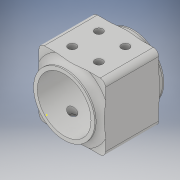
# Autodesk Inventor part: Крепление манипулятора
Saved by Autodesk Inventor 2019.1 (Build 231200000, 200)
## iProperties
Created: 2018-08-01
Part Number: Крепление манипулятора
Material: Типовые
Document SubType Name: Modeling
Designer: olege
Density: 1 g/cm^3
Appearance: По умолчанию
Author: olege
Autodesk Inventor part; units mm, degrees
ref_plane "YZ Plane" through (0, 0, 0) normal (1, 0, 0) x (0, 1, 0)
ref_plane "XZ Plane" through (0, 0, 0) normal (0, 1, 0) x (-1, 0, 0)
sketch "Эскиз1" plane through (0, 0, 0) normal (0, 0, 1) x (1, 0, 0)
  circle A0 centre (0, 0) radius 9.975
  dimension "d0" = 19.95
  constraints: 1 centre point, 1 coincident
  measures "d0" diameter of A0
extrude "Выдавливание1" add sketch "Эскиз1" along normal blind 7.1
sketch "Эскиз2" plane through (0, 0, 7.1) normal (0, 0, 1) x (1, 0, 0)
  circle A0 centre (0, 0) radius 9.975 projected
  circle A1 centre (0, 0) radius 11.5
  dimension "d3" = 23
  constraints: 1 centre point, 1 coincident
  measures "d3" diameter of A1
extrude "Выдавливание2" add sketch "Эскиз2" along normal blind 2.45 contours A0 | A1
sketch "Эскиз3" plane through (0, 0, 9.55) normal (0, 0, 1) x (1, 0, 0)
  line L0 (12.5, 12.5) -> (-12.5, 12.5)
  line L1 (-12.5, 12.5) -> (-12.5, -12.5)
  line L2 (-12.5, -12.5) -> (12.5, -12.5)
  line L3 (12.5, -12.5) -> (12.5, 12.5)
  line L4 (12.5, 12.5) -> (-12.5, -12.5) construction
  line L5 (-12.5, 12.5) -> (12.5, -12.5) construction
  point P0 (0, 0)
  dimension "d6" = 25
  dimension "d7" = 25
  constraints: 12 end point, 2 midpoint, 2 parallel, 1 horizontal, 1 perpendicular
  measures "d6" distance of L2.end L1.end
  measures "d7" distance of L1.end L0.end
extrude "Выдавливание3" add sketch "Эскиз3" along normal blind 20
fillet "Сопряжение1" radius 2.5 1 edges at (-11.5, 0, 9.55)
sketch "Эскиз4" plane through (0, 0, 29.55) normal (0, 0, 1) x (1, 0, 0)
  circle A0 centre (0, 0) radius 11.5
  dimension "d12" = 23
  constraints: 1 centre point, 1 coincident
  measures "d12" diameter of A0
extrude "Выдавливание4" add sketch "Эскиз4" along normal blind 2.5
sketch "Эскиз5" plane through (0, 0, 32.05) normal (0, 0, 1) x (1, 0, 0)
  circle A0 centre (0, 0) radius 9.975
  dimension "d15" = 19.95
  constraints: 1 centre point, 1 coincident
  measures "d15" diameter of A0
extrude "Выдавливание5" add sketch "Эскиз5" along normal blind 7.1
fillet "Сопряжение3" radius 2.5 1 edges at (-11.5, 0, 29.55)
fillet "Сопряжение4" radius 2 4 edges at (-12.5, -12.5, 19.55) (-12.5, 12.5, 19.55) (12.5, 12.5, 19.55) (12.5, -12.5, 19.55)
sketch "Эскиз6" plane through (0, 0, 39.15) normal (0, 0, 1) x (1, 0, 0)
  line L0 (-4, -4) -> (4, -4)
  line L1 (4, -4) -> (4, 4)
  line L2 (4, 4) -> (-4, 4)
  line L3 (-4, 4) -> (-4, -4)
  line L4 (-4, -4) -> (4, 4) construction
  line L5 (4, -4) -> (-4, 4) construction
  point P0 (0, 0)
  dimension "d20" = 8
  dimension "d21" = 8
  constraints: 12 end point, 2 midpoint, 2 parallel, 1 horizontal, 1 perpendicular
  measures "d20" distance of L2.end L1.end
  measures "d21" distance of L1.end L0.end
extrude "Выдавливание6" cut sketch "Эскиз6" against normal blind 8
sketch "Эскиз7" plane through (0, 0, 31.15) normal (0, 0, 1) x (1, 0, 0)
  circle A0 centre (0, 0) radius 1.25
  dimension "d24" = 2.5
  constraints: 1 centre point, 1 coincident
  measures "d24" diameter of A0
extrude "Выдавливание7" cut sketch "Эскиз7" against normal blind 6
sketch "Эскиз8" plane through (0, 0, 0) normal (0, 0, -1) x (-1, 0, 0)
  circle A0 centre (0, 7.5) radius 1.25
  circle A1 centre (0, -7.5) radius 1.25
  point P0 (0, 0)
  dimension "d27" = 2.5
  dimension "d28" = 2.5
  dimension "d29" = 7.5
  dimension "d30" = 7.5
  constraints: 2 centre point, 2 vertical alignment
  measures "d27" diameter of A0
  measures "d28" diameter of A1
  measures "d29" distance of point (0, 0) A1.centre
  measures "d30" distance of point (0, 0) A0.centre
extrude "Выдавливание8" cut sketch "Эскиз8" against normal blind 12
ref_plane "РабПлоскость1" through (-5.6789, -12.5, 7.55) normal (0, -1, 0) x (1, 0, 0)
sketch "Эскиз9" plane through (-5.6789, -12.5, 7.55) normal (0, -1, 0) x (1, 0, 0)
  line L0 (-4.8211, 12) -> (16.1789, 12) construction
  line L1 (10.6789, 7) -> (0.6789, 7) construction
  line L2 (0.6789, 7) -> (0.6789, 17) construction
  line L3 (0.6789, 17) -> (10.6789, 17) construction
  line L4 (10.6789, 17) -> (10.6789, 7) construction
  line L5 (10.6789, 7) -> (0.6789, 17) construction
  line L6 (0.6789, 7) -> (10.6789, 17) construction
  circle A0 centre (0.6789, 17) radius 1.5
  circle A1 centre (10.6789, 17) radius 1.5
  circle A2 centre (10.6789, 7) radius 1.5
  circle A3 centre (0.6789, 7) radius 1.5
  point P0 (5.6789, -7.55)
  point P1 (5.6789, 12)
  dimension "d33" = 10
  dimension "d34" = 10
  dimension "d35" = 3
  dimension "d36" = 3
  dimension "d37" = 3
  dimension "d38" = 3
  constraints: 14 end point, 4 centre point, 4 coincident, 2 midpoint, 2 parallel, 1 horizontal, 1 perpendicular
  measures "d33" distance of L2.end L3.end
  measures "d34" distance of L1.end L2.end
  measures "d35" diameter of A0
  measures "d36" diameter of A1
  measures "d37" diameter of A2
  measures "d38" diameter of A3
extrude "Выдавливание9" cut sketch "Эскиз9" against normal blind 41.975
sketch "Эскиз10" plane through (0, 0, 39.15) normal (0, 0, 1) x (1, 0, 0)
  point P0 (0, 0)
sketch "Эскиз11" plane through (0, 0, 39.15) normal (0, 0, 1) x (1, 0, 0)
  circle A0 centre (0, 0) radius 1.25 construction
  circle A1 centre (0, 0) radius 8.5 construction
  circle A2 centre (-8.5, 0) radius 1.25
  circle A3 centre (0, 8.5) radius 1.25
  circle A4 centre (8.5, 0) radius 1.25
  circle A5 centre (0, -8.5) radius 1.25
  dimension "d44" = 17
  dimension "d45" = 2.5
  dimension "d46" = 2.5
  dimension "d47" = 2.5
  dimension "d48" = 2.5
  constraints: 5 centre point, 4 point on circle, 1 coincident
  measures "d44" diameter of A1
  measures "d45" diameter of A2
  measures "d46" diameter of A3
  measures "d47" diameter of A4
  measures "d48" diameter of A5
extrude "Выдавливание10" cut sketch "Эскиз11" against normal blind 12
sketch "Эскиз12" plane through (0, 0, 39.15) normal (0, 0, 1) x (1, 0, 0)
  circle A0 centre (0, 8.5) radius 1.25 projected
  line L0 (-1.25, 8.5) -> (-1.25, 10.8162)
  line L1 (-1.25, 10.8162) -> (1.25, 10.8162)
  line L2 (1.25, 10.8162) -> (1.25, 8.5)
  line L3 (1.25, 8.5) -> (-1.25, 8.5)
  point P0 (0, 0)
  point P1 (0, 10)
  constraints: 8 end point, 3 vertical, 2 perpendicular, 3 other
extrude "Выдавливание11" cut sketch "Эскиз12" against normal up to surface (7.1 mm away) contours L3 A0 | A0 L0 L1 L2 picked at (0.0502, 8.9136)
fillet "Сопряжение5" radius 1 2 edges at (-1.25, 9.8964, 35.6) (1.25, 9.8964, 35.6)
pattern_circular "Круговой массив1" count 4 over 360 about axis through (0, 0, 32.05) along (0, 0, 1) of "Выдавливание11", "Сопряжение5"
chamfer "Фаска2" distance 2 angle 45 4 edges at (-6.5, -12.5, 24.55) (-6.5, -12.5, 14.55) (3.5, -12.5, 14.55) (3.5, -12.5, 24.55)
sketch "Эскиз13" plane through (0, 0, 32.05) normal (0, 0, 1) x (1, 0, 0)
  circle A0 centre (0, 0) radius 10.6392
  constraints: 1 centre point, 1 coincident
extrude "Выдавливание12" cut sketch "Эскиз13" along normal blind 10
sketch "Эскиз14" plane through (0, 0, 31.15) normal (0, 0, 1) x (1, 0, 0)
  circle A0 centre (0, 0) radius 1.25 projected
  line L0 (4, -4) -> (-4, -4) projected
  line L1 (4, 4) -> (4, -4) projected
  line L2 (-4, 4) -> (4, 4) projected
  line L3 (-4, -4) -> (-4, 4) projected
extrude "Выдавливание13" add sketch "Эскиз14" along normal up to surface (0.9 mm away)
sketch "Эскиз15" plane through (0, 0, 25.15) normal (0, 0, 1) x (1, 0, 0)
  circle A0 centre (0, 0) radius 1.25 projected
  circle A1 centre (-8.5, 0) radius 1.25 projected
  circle A2 centre (0, 8.5) radius 1.25 projected
  circle A3 centre (8.5, 0) radius 1.25 projected
  circle A4 centre (0, -8.5) radius 1.25 projected
extrude "Выдавливание14" add sketch "Эскиз15" along normal up to surface (6.9 mm away)
sketch "Эскиз16" plane through (0, 0, 0) normal (0, 0, -1) x (-1, 0, 0)
  circle A0 centre (0, 0) radius 18.4377
  constraints: 1 centre point, 1 coincident
extrude "Выдавливание15" cut sketch "Эскиз16" against normal up to surface (7.1 mm away)
sketch "Эскиз17" plane through (0, 7.5, 12) normal (0, 0, -1) x (-1, 0, 0)
  circle A0 centre (0, 0) radius 1.25 projected
  circle A1 centre (0, -15) radius 1.25 projected
  point P0 (0, -7.5)
extrude "Выдавливание16" add sketch "Эскиз17" along normal up to surface (4.9 mm away)
sketch "Эскиз18" plane through (0, 0, 7.1) normal (0, 0, -1) x (-1, 0, 0)
  circle A0 centre (0, 0) radius 10.1
  dimension "d70" = 20.2
  constraints: 1 centre point, 1 coincident
  measures "d70" diameter of A0
extrude "Выдавливание17" cut sketch "Эскиз18" against normal blind 29.05
sketch "Эскиз19" plane through (0, 0, 32.05) normal (0, 0, 1) x (1, 0, 0)
  circle A0 centre (0, 0) radius 10.1 projected
  circle A1 centre (0, 0) radius 11.5 projected
extrude "Выдавливание18" add sketch "Эскиз19" along normal blind 0.525
sketch "Эскиз20" plane through (0, 0, 7.1) normal (0, 0, -1) x (-1, 0, 0)
  circle A0 centre (0, 0) radius 10.1 projected
  circle A1 centre (0, 0) radius 11.5 projected
extrude "Выдавливание19" add sketch "Эскиз20" along normal blind 0.525
equation "\"d30\" = d29"
equation "\"d45\" = d48"
equation "\"d47\" = d46"
equation "\"d48\" = d47"
